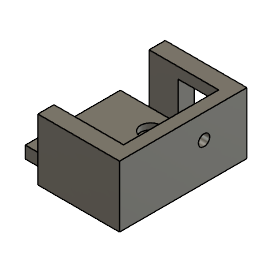
Davinki Bicep Base (Autodesk Fusion 360 design; units mm, degrees)
part number: 2026-08-31-16-49-37-012
Autodesk Fusion 360 part; units mm, degrees
note: some values were not read from the file. Chosen so that the rebuilt part matches the saved one: which bodies a step acts on; which face or edge a step refers to. Set by a fixed rule: which sketch regions a step uses.
sketch "Sketch1" plane through (0, 0, 0) normal (0, 1, 0) x (1, 0, 0)
  line L0 (0, 0) -> (0, 23.5)
  line L1 (0, 23.5) -> (-24.3, 23.5)
  line L2 (0, 0) -> (-24.3, 0)
  line L3 (-24.3, 23.5) -> (-24.3, 0)
  line L4 (0, 23.5) -> (0, 27.5)
  line L5 (0, 27.5) -> (-17.2, 27.5)
  line L6 (-17.2, 27.5) -> (-17.2, 23.5)
  line L7 (0, 0) -> (0, -4)
  line L8 (0, -4) -> (-17.2, -4)
  line L9 (-17.2, -4) -> (-17.2, 0)
  circle A0 centre (-11.8, 18.5) radius 1.125
  line L10 (0, 27.5) -> (3, 27.5)
  line L11 (0, -4) -> (3, -4)
  line L12 (3, -4) -> (3, 27.5)
  circle A1 centre (-11.8, 18.5) radius 2.475
  dimension "d2" = 23.5
  dimension "d3" = 24.3
  dimension "d4" = 24.3
  dimension "d12" = 4
  dimension "d13" = 17.2
  dimension "d14" = 4
  dimension "d15" = 17.2
  dimension "d16" = 2.25
  dimension "d17" = 3
  dimension "d18" = 3
  dimension "d59" = 4.95
  constraint coincident L0.start L2.start
  constraint vertical L0
  constraint perpendicular L0 L1
  constraint perpendicular L0 L2
  constraint perpendicular L1 L4
  constraint perpendicular L4 L5
  constraint coincident L1 L6.end
  constraint perpendicular L1 L6
  constraint perpendicular L2 L7
  constraint perpendicular L0 L8
  constraint coincident L2 L9.end
  constraint perpendicular L2 L9
  constraint perpendicular L4 L10
  constraint perpendicular L7 L11
  constraint concentric A0 A1
  measures "d2" distance of L0.start L0.end
  measures "d3" distance of L0.end L1.end
  measures "d4" distance of L0.start L2.end
  measures "d12" distance of L0.end L4.end
  measures "d13" distance of L4.end L5.end
  measures "d14" distance of L0.start L7.end
  measures "d15" distance of L7.end L8.end
  measures "d16" diameter of A0
  measures "d17" distance of L4.end L10.end
  measures "d18" distance of L7.end L11.end
  measures "d59" diameter of A1
extrude "Extrude1" add sketch "Sketch1" along normal blind 3 contours L0 L1 L2 L3 | L2 L7 L8 L9 | L0 L4 L7 L10 L11 L12 | L1 L4 L5 L6 | A0 | A1 makes body 1
extrude "Extrude2" add sketch "Sketch1" along normal blind 15.2 contours L2 L7 L8 L9 | L0 L4 L7 L10 L11 L12 | L1 L4 L5 L6 bodies 1
extrude "Extrude3" add sketch "Sketch1" along normal blind 2 contours A1 bodies 1
extrude "Extrude4" cut sketch "Sketch1" along normal blind 1 contours A1 bodies 1
sketch "Sketch2" plane through (-17.2, 0, 0) normal (-1, 0, 0) x (0, 0, 1)
  line L0 (0, 0) -> (4, 0)
  line L1 (4, 0) -> (4, 15.2)
  line L2 (4, 15.2) -> (0, 15.2)
  line L3 (0, 15.2) -> (0, 3)
  line L4 (0, 3) -> (0, 0)
  circle A0 centre (2, 9.1) radius 1
  dimension "d29" = 2
  measures "d29" diameter of A0
hole "Hole1" at (-17.2, 9.1, 2) direction (1, 0, 0) diameter 2.076 depth 3 tip angle 180 bodies 1
thread "Thread1" "ISO Metric profile 2.5 M2.5x0.45 M2.5x0.45 6H" thread offset 0 thread depth 7.4
sketch "Sketch3" plane through (-17.2, 0, 0) normal (-1, 0, 0) x (0, 0, 1)
  line L0 (-27.5, 0) -> (-23.5, 0)
  line L1 (-23.5, 0) -> (-23.5, 3)
  line L2 (-23.5, 3) -> (-23.5, 15.2)
  line L3 (-23.5, 15.2) -> (-27.5, 15.2)
  line L4 (-27.5, 15.2) -> (-27.5, 0)
  line L5 (-23.5, 3) -> (-23.5, 9.1)
  line L6 (-23.5, 9.1) -> (-25.5, 9.1)
  dimension "d35" = 6.1
  dimension "d36" = 2
  constraint coincident L1.end L2.start
  constraint perpendicular L3 L5
  constraint perpendicular L4 L6
  measures "d35" distance of L1.end L5.end
  measures "d36" distance of L5.end L6.end
hole "Hole2" at (-17.2, 9.1, -25.5) direction (1, 0, 0) diameter 2.076 depth 3 tip angle 180 bodies 1
thread "Thread2" "ISO Metric profile 2.5 M2.5x0.45 M2.5x0.45 6H" thread offset 0 thread depth 7.4
sketch "Sketch4" plane through (0, 0, -27.5) normal (0, 0, -1) x (-1, 0, 0)
  line L0 (-3, 0) -> (17.2, 0)
  line L1 (17.2, 0) -> (17.2, 15.2)
  line L2 (17.2, 15.2) -> (-3, 15.2)
  line L3 (-3, 15.2) -> (-3, 0)
  line L4 (0.5, 12.5) -> (10, 12.5)
  line L5 (10, 12.5) -> (10, 2.5)
  line L6 (10, 2.5) -> (0.5, 2.5)
  line L7 (0.5, 2.5) -> (0.5, 12.5)
  constraint horizontal L4
  constraint vertical L5
  constraint horizontal L6
  constraint vertical L7
extrude "Extrude5" cut sketch "Sketch4" against normal blind 5 contours L4 L5 L6 L7 bodies 1
extrude "Extrude6" cut sketch "Sketch1" along normal blind 18 contours A1 bodies 1 makes body 2 at (-8.3653, 0, -4.0654)
extrude "Extrude7" add sketch "Sketch1" along normal blind 1 contours A1 bodies 1 2
move_face "MoveFace1" by (0, 0.5, 0) 1 faces at (-9.7884, 1, -18.3211) on bodies 1
extrude "Extrude8" cut sketch "Sketch1" along normal blind 1 contours A1 bodies 1
extrude "Extrude9" cut 1 faces at (-12.0749, 3, -18.2449) along direction (0, -1, 0) blind 11.8 on bodies 1 bodies 1
sketch "Sketch5" plane through (3, 0, 0) normal (1, 0, 0) x (0, 0, -1)
  line L0 (-4, 0) -> (27.5, 0)
  line L1 (27.5, 0) -> (27.5, 15.2)
  line L2 (27.5, 15.2) -> (-4, 15.2)
  line L3 (-4, 15.2) -> (-4, 0)
  line L4 (7.5, 0) -> (7.5, 3)
  line L5 (7.5, 3) -> (-4, 3)
  line L6 (0, 3) -> (0, 9.25)
  line L7 (0, 9.25) -> (16.9, 9.25)
  dimension "d53" = 3
  dimension "d54" = 6.25
  dimension "d55" = 16.9
  constraint coincident L0 L4.start
  constraint perpendicular L0 L4
  constraint coincident L3 L5.end
  constraint perpendicular L3 L5
  constraint coincident L5 L6.start
  constraint perpendicular L5 L6
  constraint perpendicular L6 L7
  measures "d53" distance of L4.start L4.end
  measures "d54" distance of L6.start L6.end
  measures "d55" distance of L6.end L7.end
hole "Hole3" at (3, 9.25, -16.9) direction (-1, 0, 0) diameter 2.8 depth 2.5 tip angle 180 bodies 1
